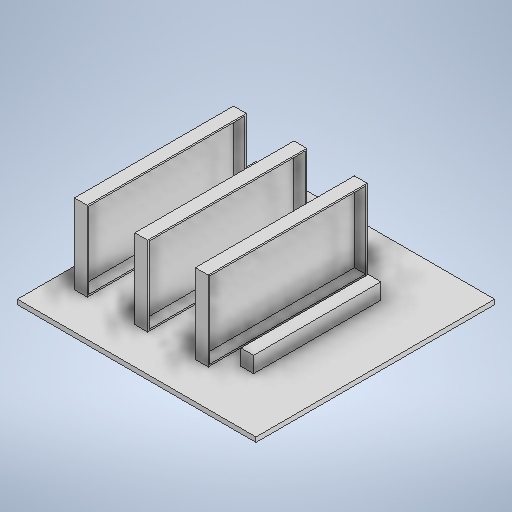
# Autodesk Inventor part: suportev2
Saved by Autodesk Inventor 2025.2 (Build 292293000, 293)
## iProperties
Created: 2025-01-27
Part Number: suportev2
Material: Genérico
Document SubType Name: Modeling
Designer: Carlos Dias
Density: 1 g/cm^3
Appearance: Padrão
Author: Carlos Dias
Autodesk Inventor part; units mm, degrees
ref_plane "YZ Plane" through (0, 0, 0) normal (1, 0, 0) x (0, 1, 0)
ref_plane "XZ Plane" through (0, 0, 0) normal (0, 1, 0) x (-1, 0, 0)
ref_plane "XY Plane" through (0, 0, 0) normal (0, 0, 1) x (1, 0, 0)
sketch "Esboço1" plane through (0, 0, 0) normal (0, 1, 0) x (-1, 0, 0)
  line L0 (75, 75) -> (-75, 75)
  line L1 (-75, 75) -> (-75, -75)
  line L2 (-75, -75) -> (75, -75)
  line L3 (75, -75) -> (75, 75)
  line L4 (75, 75) -> (-75, -75) construction
  line L5 (-75, 75) -> (75, -75) construction
  line L6 (62.1935, 51.9341) -> (54.1935, 51.9341)
  line L7 (54.1935, 51.9341) -> (54.1935, -48.0659)
  line L8 (54.1935, -48.0659) -> (62.1935, -48.0659)
  line L9 (62.1935, -48.0659) -> (62.1935, 51.9341)
  line L10 (24.1935, 51.9341) -> (16.1935, 51.9341)
  line L11 (16.1935, 51.9341) -> (16.1935, -48.0659)
  line L12 (16.1935, -48.0659) -> (24.1935, -48.0659)
  line L13 (24.1935, -48.0659) -> (24.1935, 51.9341)
  line L14 (-13.8065, 51.9341) -> (-21.8065, 51.9341)
  line L15 (-21.8065, 51.9341) -> (-21.8065, -48.0659)
  line L16 (-21.8065, -48.0659) -> (-13.8065, -48.0659)
  line L17 (-13.8065, -48.0659) -> (-13.8065, 51.9341)
  line L18 (-31.8065, 41.3063) -> (-39.8065, 41.3063)
  line L19 (-39.8065, 41.3063) -> (-39.8065, -38.6937)
  line L20 (-39.8065, -38.6937) -> (-31.8065, -38.6937)
  line L21 (-31.8065, -38.6937) -> (-31.8065, 41.3063)
  point P0 (0, 0)
  dimension "d0" = 150
  dimension "d1" = 150
  constraints: 44 end point, 10 parallel, 5 horizontal, 5 perpendicular, 2 midpoint
  measures "d0" distance of L2.end L1.end
  measures "d1" distance of L1.end L0.end
extrude "Extrusão1" add sketch "Esboço1" against normal blind 3
extrude "Extrusão2" add sketch "Esboço1" along normal blind 50 contours L9 L8 L7 L6 | L13 L12 L11 L10 | L17 L16 L15 L14
extrude "Extrusão3" add sketch "Esboço1" along normal blind 10 contours L21 L20 L19 L18
shell "Casca1" thickness 1 removed faces 3 at (21.8065, 16.6667, 18.6008) at (-16.1935, 16.6667, 18.6008) at (-54.1935, 16.6667, 18.6008)
